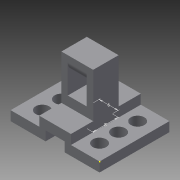
# Autodesk Inventor part: ClawAttach
Saved by Autodesk Inventor 2015 (Build 190159000, 159)
## iProperties
Created: 2016-04-06
Part Number: ClawAttach
Material: Generic
Document SubType Name: Modeling
Designer: Hatch
Density: 1 g/cm^3
Appearance: Default
Author: Hatch
Autodesk Inventor part; units mm, degrees
ref_plane "YZ Plane" through (0, 0, 0) normal (1, 0, 0) x (0, 1, 0)
ref_plane "XZ Plane" through (0, 0, 0) normal (0, 1, 0) x (-1, 0, 0)
ref_plane "XY Plane" through (0, 0, 0) normal (0, 0, 1) x (1, 0, 0)
sketch "Sketch1" plane through (0, 0, 0) normal (0, 1, 0) x (-1, 0, 0)
  line L0 (0, 0) -> (28, 0)
  line L1 (28, 0) -> (28, -22)
  line L2 (28, -22) -> (0, -22)
  line L3 (0, -22) -> (0, 0)
  dimension "d0" = 28
  dimension "d1" = 22
  constraints: 8 end point, 2 parallel, 1 horizontal, 1 perpendicular
  measures "d0" distance of L1.end L2.end
  measures "d1" distance of L0.end L1.end
extrude "Extrusion1" add sketch "Sketch1" along normal blind 3
sketch "Sketch2" plane through (0, 3, 0) normal (0, 1, 0) x (1, 0, 0)
  line L0 (-17, 7) -> (-11, 7)
  line L1 (-11, 7) -> (-11, 15)
  line L2 (-11, 15) -> (-17, 15)
  line L3 (-17, 15) -> (-17, 7)
  line L4 (-17, 7) -> (-11, 15) construction
  line L5 (-11, 7) -> (-17, 15) construction
  point P0 (0, 0)
  point P1 (-14, 11)
  dimension "d4" = 6
  dimension "d5" = 8
  constraints: 12 end point, 2 midpoint, 2 parallel, 1 horizontal, 1 perpendicular
  measures "d4" distance of L2.end L1.end
  measures "d5" distance of L1.end L0.end
sketch "Sketch3" plane through (0, 3, 0) normal (0, 1, 0) x (1, 0, 0)
  line L0 (-28, 22) -> (-28, 0) projected
  line L1 (-28, 11) -> (-23, 11)
  line L2 (0, 0) -> (0, 22) projected
  line L3 (0, 11) -> (-5, 11)
  circle A0 centre (-5, 11) radius 2.125
  dimension "d6" = 5
  dimension "d7" = 5
  dimension "d8" = 4.25
  constraints: 4 end point, 2 horizontal, 2 midpoint, 1 centre point, 1 coincident
  measures "d6" distance of L1.start L1.end
  measures "d7" distance of L3.start L3.end
  measures "d8" diameter of A0
extrude "Extrusion2" cut sketch "Sketch3" against normal through all
pattern_linear "Rectangular Pattern1" count 3 spacing 6 along (0, 0, 1) count 2 spacing 18 along (-1, 0, 0) of "Extrusion2" first direction both ways yes
sketch "Sketch5" plane through (0, 3, 0) normal (0, 1, 0) x (1, 0, 0)
  line L0 (0, 22) -> (-28, 22) projected
  line L1 (-19, 0) -> (-9, 0)
  line L2 (-9, 0) -> (-9, 22)
  line L3 (-9, 22) -> (-19, 22)
  line L4 (-19, 22) -> (-19, 0)
  line L5 (-19, 0) -> (-9, 22) construction
  line L6 (-9, 0) -> (-19, 22) construction
  point P0 (0, 0)
  point P1 (-14, 11)
  dimension "d17" = 10
  constraints: 12 end point, 2 midpoint, 2 parallel, 1 horizontal, 1 perpendicular, 1 point on line
  measures "d17" distance of L3.end L2.end
extrude "Extrusion3" add sketch "Sketch5" along normal blind 15
sketch "Sketch6" plane through (-28, 0, 0) normal (0, 0, 1) x (1, 0, 0)
  line L0 (19, 3) -> (17, 3)
  line L1 (9, 3) -> (9, 18) projected
  line L2 (9, 3) -> (11, 3)
  line L3 (0, 0) -> (28, 0) projected
  line L4 (17, 3) -> (11, 3)
  line L5 (11, 3) -> (11, 0)
  line L6 (11, 0) -> (17, 0)
  line L7 (17, 0) -> (17, 3)
  dimension "d20" = 2
  dimension "d21" = 2
  constraints: 12 end point, 2 horizontal, 2 parallel, 2 perpendicular, 1 point on line
  measures "d20" distance of L0.start L0.end
  measures "d21" distance of L1.start L2.end
extrude "Extrusion4" cut sketch "Sketch6" against normal through all
sketch "Sketch7" plane through (-9, 3, 0) normal (1, 0, 0) x (0, 0, -1)
  line L0 (0, 15) -> (7, 15)
  line L1 (22, 15) -> (0, 15) projected
  line L2 (22, 15) -> (15, 15)
  line L3 (0, 0) -> (0, 15) projected
  line L4 (7, 15) -> (0, 15)
  line L5 (0, 15) -> (0, 3)
  line L6 (0, 3) -> (7, 3)
  line L7 (7, 3) -> (7, 15)
  line L8 (22, 15) -> (15, 15)
  line L9 (15, 15) -> (15, 3)
  line L10 (15, 3) -> (22, 3)
  line L11 (22, 3) -> (22, 15)
  point P0 (0, -3)
  dimension "d24" = 7
  dimension "d25" = 7
  dimension "d26" = 12
  constraints: 20 end point, 4 parallel, 4 point on line, 2 horizontal, 2 perpendicular
  measures "d24" distance of L0.start L0.end
  measures "d25" distance of L1.start L2.end
  measures "d26" distance of L5.end L4.end
extrude "Extrusion5" cut sketch "Sketch7" against normal through all
sketch "Sketch8" plane through (-9, 6, -15) normal (0, 0, -1) x (-1, 0, 0)
  line L0 (0, 12) -> (10, 12) projected
  line L1 (5, 12) -> (5, 6)
  line L2 (10, 12) -> (10, 0) projected
  line L3 (10, 6) -> (6, 6)
  line L4 (0, 0) -> (0, 12) projected
  line L5 (0, 6) -> (4, 6)
  line L6 (2, 3) -> (8, 3)
  line L7 (8, 3) -> (8, 9)
  line L8 (8, 9) -> (2, 9)
  line L9 (2, 9) -> (2, 3)
  line L10 (2, 3) -> (8, 9) construction
  line L11 (8, 3) -> (2, 9) construction
  point P0 (-9, -6)
  dimension "d29" = 6
  dimension "d30" = 4
  dimension "d31" = 4
  constraints: 18 end point, 5 midpoint, 3 horizontal, 2 parallel, 1 perpendicular, 1 vertical
  measures "d29" distance of L1.start L1.end
  measures "d30" distance of L3.start L3.end
  measures "d31" distance of L5.start L5.end
extrude "Extrusion6" cut sketch "Sketch8" against normal through all contours L8 L7 L6 L9
fillet "Fillet1" radius 3 1 edges at (-14, 15, -7)
fillet "Fillet2" radius 3 1 edges at (-14, 15, -15)
sketch "Sketch9" plane through (0, 18, 0) normal (0, 1, 0) x (1, 0, 0)
  line L0 (-9, 7) -> (-19, 7)
  line L1 (-19, 7) -> (-19, 15)
  line L2 (-19, 15) -> (-9, 15)
  line L3 (-9, 15) -> (-9, 7)
  line L4 (-9, 7) -> (-19, 15) construction
  line L5 (-19, 7) -> (-9, 15) construction
  point P0 (0, 0)
  point P1 (-14, 11)
  constraints: 12 end point, 2 midpoint, 2 parallel, 1 horizontal, 1 perpendicular
extrude "Extrusion7" add sketch "Sketch9" along normal blind 2
body "Solid1"
